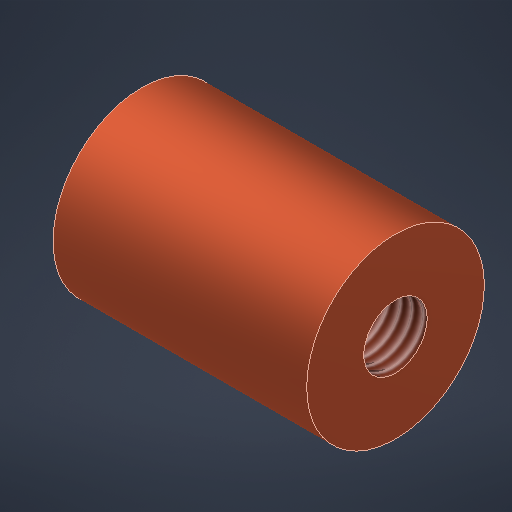
# Autodesk Inventor part: Bush_Phase
Saved by Autodesk Inventor 2026.2 (Build 302298000, 298)
## iProperties
Created: 2026-02-11
Part Number: Bush_Phase
Material: Медь
Document SubType Name: Modeling
Designer: EV-TECH
Density: 8.94 g/cm^3
Appearance: Медь — сатинированная
Author: EV-TECH
Autodesk Inventor part; units mm, degrees
ref_plane "YZ Plane" through (0, 0, 0) normal (1, 0, 0) x (0, 1, 0)
ref_plane "XZ Plane" through (0, 0, 0) normal (0, 1, 0) x (-1, 0, 0)
ref_plane "XY Plane" through (0, 0, 0) normal (0, 0, 1) x (1, 0, 0)
sketch "Эскиз1" plane through (0, 0, 0) normal (1, 0, 0) x (0, 1, 0)
  circle A0 centre (0, 0) radius 3.5
  dimension "d0" = 7
  constraints: 1 centre point, 1 coincident
  measures "d0" diameter of A0
extrude "Выдавливание1" add sketch "Эскиз1" along normal blind 10
sketch "Эскиз2" plane through (0, 0, 0) normal (-1, 0, 0) x (0, 0, 1)
  circle A0 centre (0, 0) radius 0.6
  dimension "d3" = 1.2
  constraints: 1 centre point, 1 coincident
  measures "d3" diameter of A0
extrude "Выдавливание2" add sketch "Эскиз2" along normal blind 1
sketch "Эскиз3" plane through (10, 0, 0) normal (1, 0, 0) x (0, 0, -1)
  circle A0 centre (0, 0) radius 0.6 projected
  circle A1 centre (0, 0) radius 1.25
  dimension "d6" = 2.5
  constraints: 1 centre point, 1 coincident
  measures "d6" diameter of A1
extrude "Выдавливание3" cut sketch "Эскиз3" against normal blind 8 contours A0 | A1
thread "Резьба1" size "M2.5x0.45" class "6H" standard "ANSI Metric M Profile" full length
